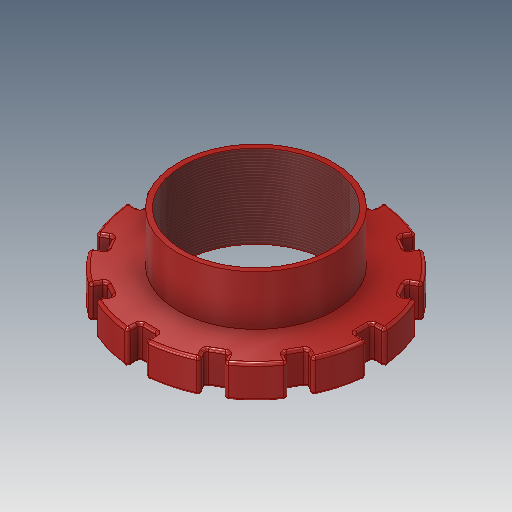
# Autodesk Inventor part: ADJUSTABLE DISC
Saved by Autodesk Inventor 2019 (Build 230136000, 136)
## iProperties
Created: 2023-06-17
Part Number: ADJUSTABLE DISC
Material: Generic
Document SubType Name: Modeling
Designer: Fransic
Density: 1 g/cm^3
Appearance: Orange-Red
Mass: 51.0353 g
Surface Area: 203.964 cm^2
Volume: 51.0353 cm^3
Author: Fransic
Autodesk Inventor part; units mm, degrees
ref_plane "YZ Plane" through (0, 0, 0) normal (1, 0, 0) x (0, 1, 0)
ref_plane "XZ Plane" through (0, 0, 0) normal (0, 1, 0) x (-1, 0, 0)
ref_plane "XY Plane" through (0, 0, 0) normal (0, 0, 1) x (1, 0, 0)
sketch "Sketch1" plane through (0, 0, 0) normal (0, 1, 0) x (-1, 0, 0)
  circle A0 centre (0, 0) radius 45
  circle A1 centre (0, 0) radius 27.5
  circle A2 centre (0, 0) radius 25
  dimension "d19" = 55
  dimension "d20" = 90
  constraints: 3 centre point, 3 coincident
  measures "d19" diameter of A1
  measures "d20" diameter of A0
extrude "Extrusion1" add sketch "Sketch1" along normal blind 12.5 contours A0
sketch "Sketch2" plane through (0, 12.5, 0) normal (0, 1, 0) x (1, 0, 0)
  circle A0 centre (0, 0) radius 25
  line L0 (0, 0) -> (-45, 0)
  circle A1 centre (0, 0) radius 45 projected
  line L1 (-24.4885, 0) -> (-38.5037, 0)
  circle A2 centre (0, 0) radius 45 projected
  line L2 (-45, -3.3195) -> (-40.2017, -3.3195)
  line L3 (-40.2017, -3.3195) -> (-40.2017, 3.3195)
  line L4 (-40.2017, 3.3195) -> (-45, 3.3195)
  line L5 (-45, 3.3195) -> (-45, -3.3195)
  dimension "d5" = 50
  constraints: 12 end point, 3 horizontal, 2 horizontal alignment, 2 parallel, 1 centre point, 1 coincident, 1 perpendicular, 1 point on line, 1 vertical, 2 other
  measures "d5" diameter of A0
extrude "Extrusion2" cut sketch "Sketch2" against normal through all contours L3 L2 A1 L0 | L0 A1 L4 L3 | L5 L4 A1 | A1 L2 L5
pattern_circular "Circular Pattern1" count 12 over 360 about axis through (0, 0, 0) along (0, 1, 0) of "Extrusion2"
fillet "Fillet1" radius 1 4 edges at (-22.9756, 6.25, 33.1559) (-17.226, 6.25, 36.4754) (-19.5639, 6.25, 40.5247) (-25.3135, 6.25, 37.2052)
pattern_circular "Circular Pattern2" count 12 over 360 about axis through (0, 0, 0) along (0, 1, 0) of "Fillet1"
thread "Thread1" size "M30x1" class "6H" standard "ANSI Metric M Profile" full length
fillet "Fillet2" radius 1 192 edges at (-44.5285, 12.5, -3.648) (-42.4946, 12.5, -3.3195) (-40.4946, 12.5, -3.0266) (-40.2017, 12.5, 0) (-40.4946, 12.5, 3.0266) (-42.4946, 12.5, 3.3195) (-44.5285, 12.5, 3.648) (-43.4667, 12.5, 11.6469) (-40.3868, 12.5, 19.1049) (-38.4611, 12.5, 18.3725) (-36.5826, 12.5, 17.6261) (-34.8157, 12.5, 20.1008) (-33.556, 12.5, 22.8684) (-35.1416, 12.5, 24.1221) (-36.7388, 12.5, 25.4235) (-31.8198, 12.5, 31.8198) (-25.4235, 12.5, 36.7388) (-24.1221, 12.5, 35.1416) (-22.8684, 12.5, 33.556) (-20.1008, 12.5, 34.8157) (-17.6261, 12.5, 36.5826) (-18.3725, 12.5, 38.4611) (-19.1049, 12.5, 40.3868) (-11.6469, 12.5, 43.4667) (-3.648, 12.5, 44.5285) (-3.3195, 12.5, 42.4946) (-3.0266, 12.5, 40.4946) (0, 12.5, 40.2017) (3.0266, 12.5, 40.4946) (3.3195, 12.5, 42.4946) (3.648, 12.5, 44.5285) (11.6469, 12.5, 43.4667) (19.1049, 12.5, 40.3868) (18.3725, 12.5, 38.4611) (17.6261, 12.5, 36.5826) (20.1008, 12.5, 34.8157) (22.8684, 12.5, 33.556) (24.1221, 12.5, 35.1416) (25.4235, 12.5, 36.7388) (31.8198, 12.5, 31.8198) (36.7388, 12.5, 25.4235) (35.1416, 12.5, 24.1221) (33.556, 12.5, 22.8684) (34.8157, 12.5, 20.1008) (36.5826, 12.5, 17.6261) (38.4611, 12.5, 18.3725) (40.3868, 12.5, 19.1049) (43.4667, 12.5, 11.6469) (44.5285, 12.5, 3.648) (42.4946, 12.5, 3.3195) (40.4946, 12.5, 3.0266) (40.2017, 12.5, 0) (40.4946, 12.5, -3.0266) (42.4946, 12.5, -3.3195) (44.5285, 12.5, -3.648) (43.4667, 12.5, -11.6469) (40.3868, 12.5, -19.1049) (38.4611, 12.5, -18.3725) (36.5826, 12.5, -17.6261) (34.8157, 12.5, -20.1008) (33.556, 12.5, -22.8684) (35.1416, 12.5, -24.1221) (36.7388, 12.5, -25.4235) (31.8198, 12.5, -31.8198) (25.4235, 12.5, -36.7388) (24.1221, 12.5, -35.1416) (22.8684, 12.5, -33.556) (20.1008, 12.5, -34.8157) (17.6261, 12.5, -36.5826) (18.3725, 12.5, -38.4611) (19.1049, 12.5, -40.3868) (11.6469, 12.5, -43.4667) (3.648, 12.5, -44.5285) (3.3195, 12.5, -42.4946) (3.0266, 12.5, -40.4946) (0, 12.5, -40.2017) (-3.0266, 12.5, -40.4946) (-3.3195, 12.5, -42.4946) (-3.648, 12.5, -44.5285) (-11.6469, 12.5, -43.4667) (-19.1049, 12.5, -40.3868) (-18.3725, 12.5, -38.4611) (-17.6261, 12.5, -36.5826) (-20.1008, 12.5, -34.8157) (-22.8684, 12.5, -33.556) (-24.1221, 12.5, -35.1416) (-25.4235, 12.5, -36.7388) (-31.8198, 12.5, -31.8198) (-36.7388, 12.5, -25.4235) (-35.1416, 12.5, -24.1221) (-33.556, 12.5, -22.8684) (-34.8157, 12.5, -20.1008) (-36.5826, 12.5, -17.6261) (-38.4611, 12.5, -18.3725) (-40.3868, 12.5, -19.1049) (-43.4667, 12.5, -11.6469) (-40.3868, 0, -19.1049) (-38.4611, 0, -18.3725) (-36.5826, 0, -17.6261) (-34.8157, 0, -20.1008) (-33.556, 0, -22.8684) (-35.1416, 0, -24.1221) (-36.7388, 0, -25.4235) (-31.8198, 0, -31.8198) (-25.4235, 0, -36.7388) (-24.1221, 0, -35.1416) (-22.8684, 0, -33.556) (-20.1008, 0, -34.8157) (-17.6261, 0, -36.5826) (-18.3725, 0, -38.4611) (-19.1049, 0, -40.3868) (-11.6469, 0, -43.4667) (-3.648, 0, -44.5285) (-3.3195, 0, -42.4946) (-3.0266, 0, -40.4946) (0, 0, -40.2017) (3.0266, 0, -40.4946) (3.3195, 0, -42.4946) (3.648, 0, -44.5285) (11.6469, 0, -43.4667) (19.1049, 0, -40.3868) (18.3725, 0, -38.4611) (17.6261, 0, -36.5826) (20.1008, 0, -34.8157) (22.8684, 0, -33.556) (24.1221, 0, -35.1416) (25.4235, 0, -36.7388) (31.8198, 0, -31.8198) (36.7388, 0, -25.4235) (35.1416, 0, -24.1221) (33.556, 0, -22.8684) (34.8157, 0, -20.1008) (36.5826, 0, -17.6261) (38.4611, 0, -18.3725) (40.3868, 0, -19.1049) (43.4667, 0, -11.6469) (44.5285, 0, -3.648) (42.4946, 0, -3.3195) (40.4946, 0, -3.0266) (40.2017, 0, 0) (40.4946, 0, 3.0266) (42.4946, 0, 3.3195) (44.5285, 0, 3.648) (43.4667, 0, 11.6469) (40.3868, 0, 19.1049) (38.4611, 0, 18.3725) (36.5826, 0, 17.6261) (34.8157, 0, 20.1008) (33.556, 0, 22.8684) (35.1416, 0, 24.1221) (36.7388, 0, 25.4235) (31.8198, 0, 31.8198) (25.4235, 0, 36.7388) (24.1221, 0, 35.1416) (22.8684, 0, 33.556) (20.1008, 0, 34.8157) (17.6261, 0, 36.5826) (18.3725, 0, 38.4611) (19.1049, 0, 40.3868) (11.6469, 0, 43.4667) (3.648, 0, 44.5285) (3.3195, 0, 42.4946) (3.0266, 0, 40.4946) (0, 0, 40.2017) (-3.0266, 0, 40.4946) (-3.3195, 0, 42.4946) (-3.648, 0, 44.5285) (-11.6469, 0, 43.4667) (-19.1049, 0, 40.3868) (-18.3725, 0, 38.4611) (-17.6261, 0, 36.5826) (-20.1008, 0, 34.8157) (-22.8684, 0, 33.556) (-24.1221, 0, 35.1416) (-25.4235, 0, 36.7388) (-31.8198, 0, 31.8198) (-36.7388, 0, 25.4235) (-35.1416, 0, 24.1221) (-33.556, 0, 22.8684) (-34.8157, 0, 20.1008) (-36.5826, 0, 17.6261) (-38.4611, 0, 18.3725) (-40.3868, 0, 19.1049) (-43.4667, 0, 11.6469) (-44.5285, 0, 3.648) (-42.4946, 0, 3.3195) (-40.4946, 0, 3.0266) (-40.2017, 0, 0) (-40.4946, 0, -3.0266) (-42.4946, 0, -3.3195) (-44.5285, 0, -3.648) (-43.4667, 0, -11.6469)
sketch "Sketch3" plane through (0, 12.5, 0) normal (0, 1, 0) x (1, 0, 0)
  circle A0 centre (0, 0) radius 29.3292
  circle A1 centre (0, 0) radius 27.5
  constraints: 2 centre point, 2 coincident
extrude "Extrusion3" add sketch "Sketch3" along normal blind 18.75
body "Solid1"
